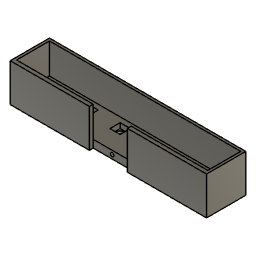
Power Supply v7 (Autodesk Fusion 360 design; units mm, degrees)
Autodesk Fusion 360 part; units mm, degrees
sketch "Schizzo1" plane through (0, 0, 0) normal (0, 0, 1) x (1, 0, 0)
  line L0 (-97.6601, 78.8336) -> (53.3399, 78.8336)
  line L1 (53.3399, 78.8336) -> (53.3399, 51.8336)
  line L2 (53.3399, 51.8336) -> (-97.6601, 51.8336)
  line L3 (-97.6601, 51.8336) -> (-97.6601, 78.8336)
  line L4 (55.3399, 49.8336) -> (-99.6601, 49.8336)
  line L5 (-99.6601, 49.8336) -> (-99.6601, 80.8336)
  line L6 (-99.6601, 80.8336) -> (55.3399, 80.8336)
  line L7 (55.3399, 80.8336) -> (55.3399, 49.8336)
  line L8 (-99.6601, 65.3336) -> (55.3399, 65.3336) construction
  line L9 (-29.8101, 66.7836) -> (-37.9101, 66.7836)
  line L10 (-37.9101, 66.7836) -> (-37.9101, 74.8836)
  line L11 (-37.9101, 74.8836) -> (-29.8101, 74.8836)
  line L12 (-29.8101, 74.8836) -> (-29.8101, 66.7836)
  line L13 (-29.8101, 66.7836) -> (-37.9101, 74.8836) construction
  line L14 (-37.9101, 66.7836) -> (-29.8101, 74.8836) construction
  circle A0 centre (-33.8601, 70.8336) radius 3.4
  circle A1 centre (-84.6601, 70.8336) radius 3.4
  line L15 (-88.7101, 66.7836) -> (-88.7101, 74.8836)
  line L16 (-80.6101, 66.7836) -> (-88.7101, 66.7836)
  line L17 (-80.6101, 74.8836) -> (-80.6101, 66.7836)
  line L18 (-88.7101, 74.8836) -> (-80.6101, 74.8836)
  circle A2 centre (-59.2601, 70.8336) radius 3.4
  line L19 (-63.3101, 66.7836) -> (-63.3101, 74.8836)
  line L20 (-55.2101, 66.7836) -> (-63.3101, 66.7836)
  line L21 (-55.2101, 74.8836) -> (-55.2101, 66.7836)
  line L22 (-63.3101, 74.8836) -> (-55.2101, 74.8836)
  circle A3 centre (-8.4601, 70.8336) radius 3.4
  line L23 (-12.5101, 66.7836) -> (-12.5101, 74.8836)
  line L24 (-4.4101, 66.7836) -> (-12.5101, 66.7836)
  line L25 (-4.4101, 74.8836) -> (-4.4101, 66.7836)
  line L26 (-12.5101, 74.8836) -> (-4.4101, 74.8836)
  circle A4 centre (16.9399, 70.8336) radius 3.4
  line L27 (12.8899, 66.7836) -> (12.8899, 74.8836)
  line L28 (20.9899, 66.7836) -> (12.8899, 66.7836)
  line L29 (20.9899, 74.8836) -> (20.9899, 66.7836)
  line L30 (12.8899, 74.8836) -> (20.9899, 74.8836)
  line L31 (-99.6601, 70.8336) -> (55.3399, 70.8336) construction
  line L32 (-97.6601, 52.8336) -> (53.3399, 52.8336)
  circle A5 centre (42.3399, 70.8336) radius 3.4
  line L33 (38.2899, 66.7836) -> (38.2899, 74.8836)
  line L34 (46.3899, 66.7836) -> (38.2899, 66.7836)
  line L35 (46.3899, 74.8836) -> (46.3899, 66.7836)
  line L36 (38.2899, 74.8836) -> (46.3899, 74.8836)
  point P0 (-33.8601, 70.8336)
  dimension "d1" = 151
  dimension "d3" = -2
  dimension "d8" = 8.1
  dimension "d9" = 8.1
  dimension "d10" = 6.8
  dimension "d13" = 25.4
  dimension "d14" = 0
  dimension "d18" = 10
  dimension "d19" = 15
  dimension "d28" = 3
  dimension "d29" = 26
  dimension "d30" = 31
  constraint horizontal L0
  constraint vertical L1
  constraint horizontal L2
  constraint vertical L3
  constraint midpoint L5 L8.start
  constraint midpoint L7 L8.end
  constraint horizontal L9
  constraint perpendicular L9 L10
  constraint parallel L9 L11
  constraint parallel L10 L12
  constraint coincident L13 P0
  constraint coincident L14 P0
  constraint coincident P0 A0.centre
  constraint coincident L5 L31.start
  constraint coincident L7 L31.end
  constraint perpendicular L7 L31
  constraint coincident P0 L31
  constraint coincident L3 L32.start
  constraint coincident L1 L32.end
  constraint perpendicular L1 L32
  measures "d1" distance of L0.start L0.end
  measures "d8" distance of L10.end L11.end
  measures "d9" distance of L9.end L10.end
  measures "d10" diameter of A0
  measures "d18" distance of L6 L31
  measures "d19" distance of L5 A1.centre
  measures "d28" distance of L4 L32
  measures "d29" distance of L0 L32
  measures "d30" distance of L4 L6
extrude "Estrusione1" add sketch "Schizzo1" along normal blind 6 contours L0 L1 L3 L32 | L1 L2 L3 L32
extrude "Estrusione3" add sketch "Schizzo1" along normal blind 2 contours L9 L10 L11 L12 | L15 L16 L17 L18 | L19 L20 L21 L22 | L23 L24 L25 L26 | L27 L28 L29 L30 | L33 L34 L35 L36
extrude "Estrusione2" add sketch "Schizzo1" along normal blind 30 contours L1 L2 L3 L32 | L4 L5 L6 L7
sketch "Schizzo2" plane through (0, 49.8336, 0) normal (0, -1, 0) x (1, 0, 0)
  line L0 (-99.6601, 0) -> (55.3399, 0)
  line L1 (55.3399, 0) -> (55.3399, 30)
  line L2 (55.3399, 30) -> (-99.6601, 30)
  line L3 (-99.6601, 30) -> (-99.6601, 0)
  line L4 (-99.6601, 30) -> (55.3399, 30) construction
  line L5 (55.3399, 30) -> (55.3399, 0) construction
  line L6 (55.3399, 0) -> (-99.6601, 0) construction
  line L7 (-99.6601, 0) -> (-99.6601, 30) construction
  line L8 (-22.1601, 30) -> (-22.1601, 0) construction
  line L9 (-99.6601, 6) -> (55.3399, 6) construction
  line L10 (-7.1601, 30) -> (-37.1601, 30)
  line L11 (-37.1601, 30) -> (-37.1601, 0)
  line L12 (-37.1601, 0) -> (-7.1601, 0)
  line L13 (-7.1601, 0) -> (-7.1601, 30)
  line L14 (-7.1601, 30) -> (-37.1601, 0) construction
  line L15 (-37.1601, 30) -> (-7.1601, 0) construction
  circle A0 centre (-22.1601, 3) radius 1.4
  point P0 (-22.1601, 15)
  dimension "d20" = 6
  dimension "d21" = 30
  dimension "d22" = 2.8
  dimension "d23" = 3
  constraint horizontal L4
  constraint vertical L5
  constraint horizontal L6
  constraint vertical L7
  constraint coincident L2.end L3.start
  constraint coincident L0.end L1.start
  constraint midpoint L4 L8.start
  constraint midpoint L6 L8.end
  constraint coincident L7 L9.start
  constraint coincident L5 L9.end
  constraint perpendicular L5 L9
  constraint horizontal L10
  constraint perpendicular L10 L11
  constraint parallel L10 L12
  constraint parallel L11 L13
  constraint coincident L14 P0
  constraint coincident L15 P0
  constraint midpoint L8 P0
  constraint collinear L4 L10
  constraint coincident L8 A0.centre
  measures "d20" distance of L6 L9
  measures "d21" distance of L11.end L12.end
  measures "d22" diameter of A0
  measures "d23" distance of L6 A0.centre
extrude "Estrusione4" cut sketch "Schizzo2" against normal blind 30 contours A0
extrude "Estrusione5" cut sketch "Schizzo2" against normal blind 3 contours L0 L2 L10 L11 L12 L13
